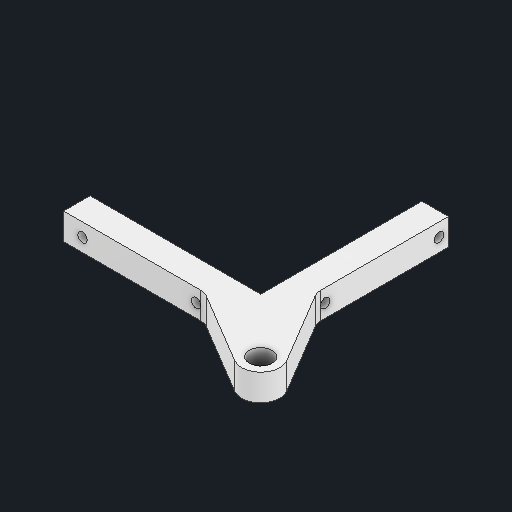
# Autodesk Inventor part: GPSholder
Saved by Autodesk Inventor 2022 (Build 260153000, 153)
## iProperties
Created: 2022-07-01
Part Number: GPSholder
Material: PC/ABS Plastic
Document SubType Name: Modeling
Designer: ForseFire
Density: 0.357273 g/cm^3
Appearance: Smooth - White
Author: ForseFire
Autodesk Inventor part; units mm, degrees
ref_plane "YZ Plane" through (0, 0, 0) normal (1, 0, 0) x (0, 1, 0)
ref_plane "XZ Plane" through (0, 0, 0) normal (0, 1, 0) x (-1, 0, 0)
ref_plane "XY Plane" through (0, 0, 0) normal (0, 0, 1) x (1, 0, 0)
sketch "Sketch1" plane through (0, 0, 0) normal (0, 1, 0) x (-1, 0, 0)
  line L0 (0, 0) -> (16.4443, 0)
  line L1 (0, 0) -> (0, -35)
  line L2 (0, -17.5) -> (0, 7.5)
  line L3 (0, 7.5) -> (45, 7.5)
  line L4 (0, -35) -> (-7, -35)
  line L5 (-7, -35) -> (-7, 14.5)
  line L6 (8.8556, 14.5) -> (45, 14.5)
  line L7 (45, 14.5) -> (45, 7.5)
  line L8 (0, 7.5) -> (-14.2941, 21.7941)
  line L9 (0, 7.5) -> (20.2149, 7.5) construction
  circle A0 centre (-14.2941, 21.7941) radius 3
  circle A1 centre (-14.2941, 21.7941) radius 5
  line L10 (-11.7387, 26.0918) -> (6.8113, 15.0619)
  arc A2 (6.8113, 15.0619) -> (8.8556, 14.5) centre (8.8556, 18.5) ccw
  line L11 (-18.5918, 19.2387) -> (-7.5619, 0.6887)
  arc A3 (-7, -1.3556) -> (-7.5619, 0.6887) centre (-11, -1.3556) ccw
  point P0 (-7, -1.3556)
  dimension "d8" = 10
  dimension "d0" = 35
  dimension "d2" = 25
  dimension "d3" = 45
  dimension "d4" = 7
  dimension "d5" = 7
  dimension "d6" = 135
  dimension "d7" = 6
  dimension "d9" = 4
  constraints: 24 end point, 4 horizontal, 4 point on circle, 4 symmetric about line, 3 centre point, 3 perpendicular, 2 coincident, 2 point on line, 2 tangent, 1 equal length, 1 midpoint, 1 vertical, 5 other
  measures "d0" distance of L0.start L1.end
  measures "d2" distance of L2.start L2.end
  measures "d3" distance of L2.end L3.end
  measures "d4" distance of L1.end L4.end
  measures "d5" distance between parallel lines of L3 L6
  measures "d6" angle of L9 L8
  measures "d7" diameter of A0
  measures "d9" radius of A2
extrude "Extrusion1" add sketch "Sketch1" along normal blind 7
sketch "Sketch2" plane through (0, 0, -35) normal (-1, 0, 0) x (0, 0, 1)
  line L0 (42.5, 0) -> (42.5, 7) projected
  line L1 (42.5, 3.5) -> (32.5, 3.5)
  line L2 (32.5, 3.5) -> (2.5, 3.5)
  circle A0 centre (32.5, 3.5) radius 1.25
  circle A1 centre (2.5, 3.5) radius 1.25
  point P0 (35, 0)
  dimension "d12" = 10
  dimension "d13" = 30
  dimension "d14" = 2.5
  dimension "d15" = 2.5
  constraints: 4 end point, 2 centre point, 2 coincident, 1 horizontal, 1 midpoint, 1 point on line
  measures "d12" distance of L1.start L1.end
  measures "d13" distance of L1.end L2.end
  measures "d14" diameter of A0
  measures "d15" diameter of A1
extrude "Extrusion2" cut sketch "Sketch2" against normal through all
sketch "Sketch3" plane through (0, 0, 7.5) normal (0, 0, -1) x (-1, 0, 0)
  line L0 (0, 0) -> (0, 7) projected
  line L1 (0, 3.5) -> (10, 3.5)
  line L2 (10, 3.5) -> (40, 3.5)
  circle A0 centre (40, 3.5) radius 1.25
  circle A1 centre (10, 3.5) radius 1.25
  dimension "d18" = 10
  dimension "d19" = 30
  dimension "d20" = 2.5
  dimension "d21" = 2.5
  constraints: 4 end point, 2 centre point, 2 coincident, 1 horizontal, 1 midpoint, 1 point on line
  measures "d18" distance of L1.start L1.end
  measures "d19" distance of L1.end L2.end
  measures "d20" diameter of A0
  measures "d21" diameter of A1
extrude "Extrusion3" cut sketch "Sketch3" against normal blind 10
body "Solid1"
